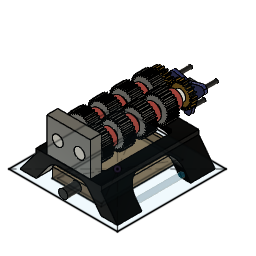
shredder_3d (Autodesk Fusion 360 design; units mm, degrees)
Autodesk Fusion 360 part; units mm, degrees
(part 1 of 2)
sketch "plane" plane through (0, 0, 0) normal (0, 0, 1) x (1, 0, 0)
  line L0 (100, 100) -> (-100, 100)
  line L1 (-100, 100) -> (-100, -100)
  line L2 (-100, -100) -> (100, -100)
  line L3 (100, -100) -> (100, 100)
  line L4 (100, 100) -> (-100, -100) construction
  line L5 (-100, 100) -> (100, -100) construction
  dimension "d1" = 200
  dimension "d2" = 200
  constraint horizontal L0
  constraint perpendicular L0 L1
  constraint parallel L0 L2
  constraint parallel L1 L3
  constraint coincident L4 origin
  constraint coincident L5 origin
  measures "d1" distance of L1.end L2.end
  measures "d2" distance of L0.end L1.end
sketch "holder" plane through (0, 0, 0) normal (0, 1, 0) x (1, 0, 0)
  line L0 (90, 0, 90) -> (60, -40, 90)
  line L1 (60, -40, 90) -> (30, -40, 90)
  line L2 (30, -40, 90) -> (60, 0, 90)
  line L3 (60, 0, 90) -> (90, 0, 90)
  line L4 (0, -30) -> (0, 30)
  line L5 (-30, -40, 90) -> (-60, 0, 90)
  line L6 (-60, -40, 90) -> (-30, -40, 90)
  line L7 (-90, 0, 90) -> (-60, -40, 90)
  line L8 (-60, 0, 90) -> (-90, 0, 90)
  line L9 (30, -40, -90) -> (60, 0, -90)
  line L10 (60, -40, -90) -> (30, -40, -90)
  line L11 (90, 0, -90) -> (60, -40, -90)
  line L12 (60, 0, -90) -> (90, 0, -90)
  line L13 (-60, 0, -90) -> (-90, 0, -90)
  line L14 (-90, 0, -90) -> (-60, -40, -90)
  line L15 (-60, -40, -90) -> (-30, -40, -90)
  line L16 (-30, -40, -90) -> (-60, 0, -90)
  constraint vertical L4
extrude "Extrude1" add sketch "holder" along normal blind 25 contours L9 L10 L11 L12 | L13 L14 L15 L16 in plane through (0, -90, 0) normal (0, 1, 0) makes body 1 at (80, -81.6667, 13.3333) makes body 2 at (-80, -81.6667, 13.3333)
extrude "Extrude2" add sketch "holder" against normal blind 25 separate body contours L0 L1 L2 L3 | L5 L6 L7 L8 in plane through (0, 90, 0) normal (0, 1, 0) makes body 3 at (-80, 81.6667, 13.3333) makes body 4 at (80, 81.6667, 13.3333)
copy_body "Body->Comp1" bodies 1 removing the originals makes body 5 in component "holder_"
copy_body "CutPasteBodies1" bodies 2 removing the originals makes body 6 in component "holder_"
copy_body "CutPasteBodies2" bodies 3 removing the originals makes body 7 in component "holder_"
copy_body "CutPasteBodies3" bodies 4 removing the originals makes body 8 in component "holder_"
sketch "holder_1" plane through (0, 65, 0) normal (0, -1, 0) x (1, 0, 0) in component "holder_"
  line L0 (-90, 0) -> (-60, 0)
  line L1 (-60, 0) -> (-30, 40)
  line L2 (-30, 40) -> (-60, 40)
  line L3 (-60, 40) -> (-90, 0)
  line L4 (-60, 40) -> (-45, 40)
  line L5 (-60, 40) -> (-40, 40)
  line L6 (-60, 40) -> (-90, 0)
  line L7 (-90, 0) -> (-70, 0)
  line L8 (-70, 0) -> (-40, 40)
  line L9 (60, 40) -> (40, 40)
  line L10 (40, 40) -> (70, 0)
  line L11 (70, 0) -> (90, 0)
  line L12 (90, 0) -> (60, 40)
  constraint coincident L2.end L3.start
  constraint midpoint L2 L4.end
  constraint coincident L2 L5.end
  constraint parallel L2 L5
  constraint coincident L0.start L3.end
  constraint coincident L0 L7.end
  constraint parallel L0 L7
  constraint parallel L6 L8
  constraint parallel L0 L9
  constraint parallel L9 L11
  constraint parallel L10 L12
extrude "Extrude1'" add sketch "holder_1" along normal blind 20 contours L0 L2 L3 L4 L5 L6 L7 L8 | L9 L10 L11 L12 bodies 8 makes body 9 at (-70, 58.3333, 26.6667) in component "holder_"
combine "Combine1" operation add target body 9 tool bodies 7 in component "holder_"
sketch "holder_2_extrude" plane through (0, -65, 0) normal (0, 1, 0) x (-1, 0, 0) in component "holder_"
  line L0 (-60, 0) -> (-30, 40)
  line L1 (-30, 40) -> (-60, 40)
  line L2 (-60, 40) -> (-90, 0)
  line L3 (-90, 0) -> (-60, 0)
  line L4 (-60, 40) -> (-40, 40)
  line L5 (-60, 40) -> (-90, 0)
  line L6 (-90, 0) -> (-70, 0)
  line L7 (-70, 0) -> (-40, 40)
  line L8 (60, 40) -> (40, 40)
  line L9 (40, 40) -> (70, 0)
  line L10 (70, 0) -> (90, 0)
  line L11 (90, 0) -> (60, 40)
  constraint coincident L1.end L2.start
  constraint coincident L1 L4.end
  constraint parallel L1 L4
  constraint coincident L2.end L3.start
  constraint coincident L3 L6.end
  constraint parallel L3 L8
  constraint parallel L8 L10
  constraint parallel L9 L11
extrude "Extrude2'" add sketch "holder_2_extrude" along normal blind 20 contours L1 L2 L3 L4 L5 L6 L7 | L8 L9 L10 L11 bodies 5 6 in component "holder_"
sketch "base" plane through (0, 0, 40) normal (0, 0, 1) x (-1, 0, 0) in component "holder_"
  line L0 (60, -90) -> (60, -45)
  line L1 (60, -45) -> (40, -45)
  line L2 (40, -45) -> (40, -65)
  line L3 (40, -65) -> (30, -65)
  line L4 (30, -65) -> (30, -90)
  line L5 (30, -90) -> (60, -90)
  line L6 (60, -90) -> (-60, -90)
  line L7 (-60, -90) -> (-60, -65)
  line L8 (-60, -65) -> (60, -65)
  line L9 (60, -65) -> (60, 90)
  line L10 (60, 90) -> (40, 90)
  line L11 (40, 90) -> (40, -65)
  line L12 (-39.8261, -65) -> (-39.8261, 90)
  line L13 (-39.8261, 90) -> (-60, 90)
  line L14 (-60, 90) -> (-60, -65)
  line L15 (40, 90) -> (-39.8261, 90)
  line L16 (40, 65.705) -> (-39.8261, 65.705)
  constraint coincident L0.start L5.end
  constraint perpendicular L0 L6
  constraint perpendicular L5 L7
  constraint coincident L0 L8.end
  constraint perpendicular L0 L8
  constraint perpendicular L8 L9
  constraint perpendicular L0 L10
  constraint coincident L2.end L3.start
  constraint perpendicular L3 L11
  constraint coincident L8 L12.start
  constraint perpendicular L8 L12
  constraint perpendicular L12 L13
  constraint perpendicular L8 L14
  constraint perpendicular L11 L15
  constraint coincident L11 L16.start
  constraint coincident L12 L16.end
  constraint perpendicular L12 L16
extrude "Extrude3" add sketch "base" along normal blind 8 contours L0 L3 L4 L5 L6 L8 | L0 L1 L2 L8 L9 L11 | L4 L6 L7 L8 | L1 L9 L10 L11 | L8 L12 L13 L14 | L11 L12 L15 L16 bodies 5 6 8 9 in component "holder_"
fillet "Fillet1" radius 24.5 8 edges at (30, 77.5, 40) (50, 45, 40) (50, -45, 40) (30, -77.8525, 40) (-50, 45, 40) (-30, 77.5, 40) (-50, -45, 40) (-30, -77.8525, 40) on bodies 5 in component "holder_"
sketch "decorative_glass" plane through (0, 45, 0) normal (0, -1, 0) x (1, 0, 0) in component "holder_"
  line L0 (78.375, 15.5) -> (58.375, 15.5)
  line L1 (58.375, 15.5) -> (70, 0)
  line L2 (70, 0) -> (90, 0)
  line L3 (90, 0) -> (78.375, 15.5)
  circle A0 centre (75.5122, 6.7743) radius 5
  circle A1 centre (-74.4878, 6.7743) radius 5
  dimension "d15" = 10
  dimension "d16" = 10
  measures "d15" diameter of A0
  measures "d16" diameter of A1
extrude "Extrude4" cut sketch "decorative_glass" along normal blind 100 and the other way blind 20 contours A0 | A1 bodies 5 in component "holder_"
chamfer "Chamfer1" distance 5 angle 45 4 edges at (39.8261, -65.705, 44) (-40, -65.705, 44) (-40, 65, 44) (39.8261, 65, 44) on bodies 5 in component "holder_"
sketch "decorative_glass (1)" plane through (0, -45, 0) normal (0, 1, 0) x (-1, 0, 0) in component "holder_"
  circle A0 centre (-75.5122, 6.7743) radius 5
  line L0 (-58.375, 15.5) -> (-78.375, 15.5)
  line L1 (-78.375, 15.5) -> (-90, 0)
  line L2 (-90, 0) -> (-70, 0)
  line L3 (-70, 0) -> (-58.375, 15.5)
  circle A1 centre (-75.5122, 6.7743) radius 4.85
  circle A2 centre (74.4878, 6.7743) radius 4.85
  dimension "d22" = 9.7
  dimension "d23" = 9.7
  constraint concentric A0 A1
  measures "d22" diameter of A1
  measures "d23" diameter of A2
extrude "Extrude5" add sketch "decorative_glass (1)" along normal blind 105 and the other way blind 5 separate body contours A1 | A2 makes body 10 at (70.6863, 25, 6.2914) makes body 11 at (-79.3137, 25, 6.2914) in component "holder_"
copy_body "Body->Comp1'" bodies 10 removing the originals makes body 12 in component "decoration"
copy_body "CutPasteBodies1'" bodies 11 removing the originals makes body 13 in component "decoration"
sketch "trashbin" plane through (0, 0, 0) normal (0, 0, 1) x (1, 0, 0)
  line L0 (45, 75) -> (-45, 75)
  line L1 (-45, 75) -> (-45, -75)
  line L2 (-45, -75) -> (45, -75)
  line L3 (45, -75) -> (45, 75)
  line L4 (45, 75) -> (-45, -75) construction
  line L5 (-45, 75) -> (45, -75) construction
  line L6 (-40.0498, -70.0498) -> (40.0498, -70.0498)
  line L7 (40.0498, -70.0498) -> (40.0498, 70.0498)
  line L8 (40.0498, 70.0498) -> (-40.0498, 70.0498)
  line L9 (-40.0498, 70.0498) -> (-40.0498, -70.0498)
  dimension "d28" = 90
  dimension "d29" = 150
  dimension "d30" = -4.9502
  constraint horizontal L0
  constraint perpendicular L0 L1
  constraint parallel L0 L2
  constraint parallel L1 L3
  constraint coincident L4 origin
  constraint coincident L5 origin
  measures "d28" distance of L1.end L2.end
  measures "d29" distance of L0.end L1.end
extrude "Extrude3'" add sketch "trashbin" along normal blind 19 separate body makes body 14
extrude "Extrude4'" add sketch "trashbin" along normal blind 5 contours L6 L7 L8 L9 bodies 14
copy_body "Body->Comp2" bodies 14 removing the originals makes body 15 in component "trashbin_removeable"
sketch "handle_sketch" plane through (0, -75, 0) normal (0, -1, 0) x (1, 0, 0) in component "trashbin_removeable"
  line L0 (-45, 0) -> (45, 0)
  line L1 (45, 0) -> (45, 19)
  line L2 (45, 19) -> (-45, 19)
  line L3 (-45, 19) -> (-45, 0)
  circle A0 centre (0, 10) radius 8.3009
extrude "Extrude1''" add sketch "handle_sketch" along normal blind 25 separate body contours A0 makes body 16 in component "trashbin_removeable"
sketch "back_wall" plane through (0, 0, 0) normal (0, 1, 0) x (1, 0, 0) in component "shredder_upperbody"
  line L0 (-40, -48.5, -70) -> (40, -48.5, -70)
  line L1 (40, -48.5, -70) -> (40, -111.5, -70)
  line L2 (40, -111.5, -70) -> (-40, -111.5, -70)
  line L3 (-40, -111.5, -70) -> (-40, -48.5, -70)
  line L4 (-40, -48.5, -70) -> (40, -111.5, -70) construction
  line L5 (40, -48.5, -70) -> (-40, -111.5, -70) construction
  line L6 (0, -111.5, -70) -> (0, -48.5, -70)
  line L7 (-40, -80, -70) -> (-20, -80, -70)
  line L8 (40, -80, -70) -> (20, -80, -70)
  circle A0 through (-10, -80, -70) (-25, -71.3397, -70) (-25, -88.6603, -70)
  circle A1 through (30, -80, -70) (15, -71.3397, -70) (15, -88.6603, -70)
  point P0 (0, -80)
  dimension "d37" = 63
  dimension "d38" = 20
extrude "Extrude1'''" add sketch "back_wall" along normal blind -20 and the other way blind 0 separate body contours L0 L2 L3 L6 | L0 L1 L2 L6 in plane through (0, -70, 0) normal (0, 1, 0) makes body 17 in component "shredder_upperbody"
sketch "pin" plane through (0, 0, 0) normal (0, 1, 0) x (1, 0, 0) in component "blades_2"
  circle A0 centre (-20, -80) radius 9.795
  dimension "d43" = 19.59
  measures "d43" diameter of A0
extrude "Extrude1''''" add sketch "pin" along normal blind 90 and the other way blind 90 separate body makes body 18 in component "blades_2"
sketch "blade_sketch" plane through (0, 90, 0) normal (0, 1, 0) x (-1, 0, 0) in component "blades_2"
  circle A0 centre (20, 80) radius 9.795
  line L0 (16.7621, 104.7894) -> (18.3025, 102.5385)
  line L1 (18.3025, 102.5385) -> (17.1562, 102.2564)
  spline S0 degree 2 poles (17.1562, 102.2564) (16.2391, 98.8702) (14.8092, 101.6787) knots 0 0 0 0.491488 0.491488 0.491488 weights 1 2.231964 1
  line L2 (14.8092, 101.6787) -> (14.1792, 102.916)
  spline S1 degree 2 poles (12.2749, 101.0655) (12.1343, 97.5602) (10.1154, 99.9801) knots 0 0 0 0.491488 0.491488 0.491488 weights 1 2.231964 1
  line L3 (10.1154, 99.9801) -> (9.2259, 101.0462)
  line L4 (11.3271, 103.4474) -> (13.3298, 101.5957)
  line L5 (13.3298, 101.5957) -> (12.2749, 101.0655)
  spline S2 degree 2 poles (7.7811, 98.8184) (8.424, 95.3697) (5.9173, 97.2796) knots 0 0 0 0.491488 0.491488 0.491488 weights 1 2.231964 1
  line L6 (5.9173, 97.2796) -> (4.8128, 98.1211)
  line L7 (6.327, 100.9296) -> (8.6915, 99.57)
  line L8 (8.6915, 99.57) -> (7.7811, 98.8184)
  spline S3 degree 2 poles (3.9, 95.6276) (5.2942, 92.4084) (2.4253, 93.7127) knots 0 0 0 0.491488 0.491488 0.491488 weights 1 2.231964 1
  line L9 (2.4253, 93.7127) -> (1.1612, 94.2873)
  line L10 (2.0125, 97.3624) -> (4.6203, 96.563)
  line L11 (4.6203, 96.563) -> (3.9, 95.6276)
  spline S4 degree 2 poles (0.8262, 91.6532) (2.9018, 88.825) (-0.1854, 89.4581) knots 0 0 0 0.491488 0.491488 0.491488 weights 1 2.231964 1
  line L12 (-0.1854, 89.4581) -> (-1.5457, 89.7371)
  line L13 (-1.4, 92.9245) -> (1.3203, 92.7254)
  line L14 (1.3203, 92.7254) -> (0.8262, 91.6532)
  spline S5 degree 2 poles (-1.2862, 87.0945) (1.3667, 84.799) (-1.784, 84.7293) knots 0 0 0 0.491488 0.491488 0.491488 weights 1 2.231964 1
  line L15 (-1.784, 84.7293) -> (-3.1722, 84.6986)
  line L16 (-3.7394, 87.8385) -> (-1.043, 88.2497)
  line L17 (-1.043, 88.2497) -> (-1.2862, 87.0945)
  spline S6 degree 2 poles (-2.3312, 82.18) (0.766, 80.5324) (-2.2902, 79.7633) knots 0 0 0 0.491488 0.491488 0.491488 weights 1 2.231964 1
  line L18 (-2.2902, 79.7633) -> (-3.6367, 79.4245)
  line L19 (-4.8884, 82.3594) -> (-2.3512, 83.3603)
  line L20 (-2.3512, 83.3603) -> (-2.3312, 82.18)
  spline S7 degree 2 poles (-2.2564, 77.1562) (1.1298, 76.2391) (-1.6787, 74.8092) knots 0 0 0 0.491488 0.491488 0.491488 weights 1 2.231964 1
  line L21 (-1.6787, 74.8092) -> (-2.916, 74.1792)
  line L22 (-4.7894, 76.7621) -> (-2.5385, 78.3025)
  line L23 (-2.5385, 78.3025) -> (-2.2564, 77.1562)
  spline S8 degree 2 poles (-1.0655, 72.2749) (2.4398, 72.1343) (0.0199, 70.1154) knots 0 0 0 0.491488 0.491488 0.491488 weights 1 2.231964 1
  line L24 (0.0199, 70.1154) -> (-1.0462, 69.2259)
  line L25 (-3.4474, 71.3271) -> (-1.5957, 73.3298)
  line L26 (-1.5957, 73.3298) -> (-1.0655, 72.2749)
  spline S9 degree 2 poles (1.1816, 67.7811) (4.6303, 68.424) (2.7204, 65.9173) knots 0 0 0 0.491488 0.491488 0.491488 weights 1 2.231964 1
  line L27 (2.7204, 65.9173) -> (1.8789, 64.8128)
  line L28 (-0.9296, 66.327) -> (0.43, 68.6915)
  line L29 (0.43, 68.6915) -> (1.1816, 67.7811)
  spline S10 degree 2 poles (4.3724, 63.9) (7.5916, 65.2942) (6.2873, 62.4253) knots 0 0 0 0.491488 0.491488 0.491488 weights 1 2.231964 1
  line L30 (6.2873, 62.4253) -> (5.7127, 61.1612)
  line L31 (2.6376, 62.0125) -> (3.437, 64.6203)
  line L32 (3.437, 64.6203) -> (4.3724, 63.9)
  spline S11 degree 2 poles (8.3468, 60.8262) (11.175, 62.9018) (10.5419, 59.8146) knots 0 0 0 0.491488 0.491488 0.491488 weights 1 2.231964 1
  line L33 (10.5419, 59.8146) -> (10.2629, 58.4543)
  line L34 (7.0755, 58.6) -> (7.2746, 61.3203)
  line L35 (7.2746, 61.3203) -> (8.3468, 60.8262)
  spline S12 degree 2 poles (12.9055, 58.7138) (15.201, 61.3667) (15.2707, 58.216) knots 0 0 0 0.491488 0.491488 0.491488 weights 1 2.231964 1
  line L36 (15.2707, 58.216) -> (15.3014, 56.8278)
  line L37 (12.1615, 56.2606) -> (11.7503, 58.957)
  line L38 (11.7503, 58.957) -> (12.9055, 58.7138)
  spline S13 degree 2 poles (17.82, 57.6688) (19.4676, 60.766) (20.2367, 57.7098) knots 0 0 0 0.491488 0.491488 0.491488 weights 1 2.231964 1
  line L39 (20.2367, 57.7098) -> (20.5755, 56.3633)
  line L40 (17.6406, 55.1116) -> (16.6397, 57.6488)
  line L41 (16.6397, 57.6488) -> (17.82, 57.6688)
  spline S14 degree 2 poles (22.8438, 57.7436) (23.7609, 61.1298) (25.1908, 58.3213) knots 0 0 0 0.491488 0.491488 0.491488 weights 1 2.231964 1
  line L42 (25.1908, 58.3213) -> (25.8208, 57.084)
  line L43 (23.2379, 55.2106) -> (21.6975, 57.4615)
  line L44 (21.6975, 57.4615) -> (22.8438, 57.7436)
  spline S15 degree 2 poles (27.7251, 58.9345) (27.8657, 62.4398) (29.8846, 60.0199) knots 0 0 0 0.491488 0.491488 0.491488 weights 1 2.231964 1
  line L45 (29.8846, 60.0199) -> (30.7741, 58.9538)
  line L46 (28.6729, 56.5526) -> (26.6702, 58.4043)
  line L47 (26.6702, 58.4043) -> (27.7251, 58.9345)
  spline S16 degree 2 poles (32.2189, 61.1816) (31.576, 64.6303) (34.0827, 62.7204) knots 0 0 0 0.491488 0.491488 0.491488 weights 1 2.231964 1
  line L48 (34.0827, 62.7204) -> (35.1872, 61.8789)
  line L49 (33.673, 59.0704) -> (31.3085, 60.43)
  line L50 (31.3085, 60.43) -> (32.2189, 61.1816)
  spline S17 degree 2 poles (36.1, 64.3724) (34.7058, 67.5916) (37.5747, 66.2873) knots 0 0 0 0.491488 0.491488 0.491488 weights 1 2.231964 1
  line L51 (37.5747, 66.2873) -> (38.8388, 65.7127)
  line L52 (37.9875, 62.6376) -> (35.3797, 63.437)
  line L53 (35.3797, 63.437) -> (36.1, 64.3724)
  spline S18 degree 2 poles (39.1738, 68.3468) (37.0982, 71.175) (40.1854, 70.5419) knots 0 0 0 0.491488 0.491488 0.491488 weights 1 2.231964 1
  line L54 (40.1854, 70.5419) -> (41.5457, 70.2629)
  line L55 (41.4, 67.0755) -> (38.6797, 67.2746)
  line L56 (38.6797, 67.2746) -> (39.1738, 68.3468)
  spline S19 degree 2 poles (41.2862, 72.9055) (38.6333, 75.201) (41.784, 75.2707) knots 0 0 0 0.491488 0.491488 0.491488 weights 1 2.231964 1
  line L57 (41.784, 75.2707) -> (43.1722, 75.3014)
  line L58 (43.7394, 72.1615) -> (41.043, 71.7503)
  line L59 (41.043, 71.7503) -> (41.2862, 72.9055)
  spline S20 degree 2 poles (42.3312, 77.82) (39.234, 79.4676) (42.2902, 80.2367) knots 0 0 0 0.491488 0.491488 0.491488 weights 1 2.231964 1
  line L60 (42.2902, 80.2367) -> (43.6367, 80.5755)
  line L61 (44.8884, 77.6406) -> (42.3512, 76.6397)
  line L62 (42.3512, 76.6397) -> (42.3312, 77.82)
  spline S21 degree 2 poles (42.2564, 82.8438) (38.8702, 83.7609) (41.6787, 85.1908) knots 0 0 0 0.491488 0.491488 0.491488 weights 1 2.231964 1
  line L63 (41.6787, 85.1908) -> (42.916, 85.8208)
  line L64 (44.7894, 83.2379) -> (42.5385, 81.6975)
  line L65 (42.5385, 81.6975) -> (42.2564, 82.8438)
  spline S22 degree 2 poles (41.0655, 87.7251) (37.5602, 87.8657) (39.9801, 89.8846) knots 0 0 0 0.491488 0.491488 0.491488 weights 1 2.231964 1
  line L66 (39.9801, 89.8846) -> (41.0462, 90.7741)
  line L67 (43.4474, 88.6729) -> (41.5957, 86.6702)
  line L68 (41.5957, 86.6702) -> (41.0655, 87.7251)
  spline S23 degree 2 poles (38.8184, 92.2189) (35.3697, 91.576) (37.2796, 94.0827) knots 0 0 0 0.491488 0.491488 0.491488 weights 1 2.231964 1
  line L69 (37.2796, 94.0827) -> (38.1211, 95.1872)
  line L70 (40.9296, 93.673) -> (39.57, 91.3085)
  line L71 (39.57, 91.3085) -> (38.8184, 92.2189)
  spline S24 degree 2 poles (35.6276, 96.1) (32.4084, 94.7058) (33.7127, 97.5747) knots 0 0 0 0.491488 0.491488 0.491488 weights 1 2.231964 1
  line L72 (33.7127, 97.5747) -> (34.2873, 98.8388)
  line L73 (37.3624, 97.9875) -> (36.563, 95.3797)
  line L74 (36.563, 95.3797) -> (35.6276, 96.1)
  spline S25 degree 2 poles (31.6532, 99.1738) (28.825, 97.0982) (29.4581, 100.1854) knots 0 0 0 0.491488 0.491488 0.491488 weights 1 2.231964 1
  line L75 (29.4581, 100.1854) -> (29.7371, 101.5457)
  line L76 (32.9245, 101.4) -> (32.7254, 98.6797)
  line L77 (32.7254, 98.6797) -> (31.6532, 99.1738)
  spline S26 degree 2 poles (27.0945, 101.2862) (24.799, 98.6333) (24.7293, 101.784) knots 0 0 0 0.491488 0.491488 0.491488 weights 1 2.231964 1
  line L78 (24.7293, 101.784) -> (24.6986, 103.1722)
  line L79 (27.8385, 103.7394) -> (28.2497, 101.043)
  line L80 (28.2497, 101.043) -> (27.0945, 101.2862)
  spline S27 degree 2 poles (22.18, 102.3312) (20.5324, 99.234) (19.7633, 102.2902) knots 0 0 0 0.491488 0.491488 0.491488 weights 1 2.231964 1
  line L81 (19.7633, 102.2902) -> (19.4245, 103.6367)
  line L82 (22.3594, 104.8884) -> (23.3603, 102.3512)
  line L83 (23.3603, 102.3512) -> (22.18, 102.3312)
  line L84 (11.3271, 103.4474) -> (14.1792, 102.916)
  line L85 (6.327, 100.9296) -> (9.2259, 101.0462)
  line L86 (2.0125, 97.3624) -> (4.8128, 98.1211)
  line L87 (-1.4, 92.9245) -> (1.1612, 94.2873)
  line L88 (-3.7394, 87.8385) -> (-1.5457, 89.7371)
  line L89 (-4.8884, 82.3594) -> (-3.1722, 84.6986)
  line L90 (-4.7894, 76.7621) -> (-3.6367, 79.4245)
  line L91 (-3.4474, 71.3271) -> (-2.916, 74.1792)
  line L92 (-0.9296, 66.327) -> (-1.0462, 69.2259)
  line L93 (2.6376, 62.0125) -> (1.8789, 64.8128)
  line L94 (7.0755, 58.6) -> (5.7127, 61.1612)
  line L95 (12.1615, 56.2606) -> (10.2629, 58.4543)
  line L96 (17.6406, 55.1116) -> (15.3014, 56.8278)
  line L97 (23.2379, 55.2106) -> (20.5755, 56.3633)
  line L98 (28.6729, 56.5526) -> (25.8208, 57.084)
  line L99 (33.673, 59.0704) -> (30.7741, 58.9538)
  line L100 (37.9875, 62.6376) -> (35.1872, 61.8789)
  line L101 (41.4, 67.0755) -> (38.8388, 65.7127)
  line L102 (43.7394, 72.1615) -> (41.5457, 70.2629)
  line L103 (44.8884, 77.6406) -> (43.1722, 75.3014)
  line L104 (44.7894, 83.2379) -> (43.6367, 80.5755)
  line L105 (43.4474, 88.6729) -> (42.916, 85.8208)
  line L106 (40.9296, 93.673) -> (41.0462, 90.7741)
  line L107 (37.3624, 97.9875) -> (38.1211, 95.1872)
  line L108 (32.9245, 101.4) -> (34.2873, 98.8388)
  line L109 (27.8385, 103.7394) -> (29.7371, 101.5457)
  line L110 (22.3594, 104.8884) -> (24.6986, 103.1722)
  line L111 (16.7621, 104.7894) -> (19.4245, 103.6367)
extrude "Extrude2''" add sketch "blade_sketch" against normal blind 20 separate body makes body 19 in component "blades_2"
fillet "Fillet1'" radius 0.5 28 edges at (-14.1792, 80, 102.916) (-19.4245, 80, 103.6367) (-24.6986, 80, 103.1722) (-29.7371, 80, 101.5457) (-34.2873, 80, 98.8388) (-38.1211, 80, 95.1872) (-41.0462, 80, 90.7741) (-42.916, 80, 85.8208) (-43.6367, 80, 80.5755) (-43.1722, 80, 75.3014) (-41.5457, 80, 70.2629) (-38.8388, 80, 65.7127) (-35.1872, 80, 61.8789) (-30.7741, 80, 58.9538) (-25.8208, 80, 57.084) (-20.5755, 80, 56.3633) (-15.3014, 80, 56.8278) (-10.2629, 80, 58.4543) (-5.7127, 80, 61.1612) (-1.8789, 80, 64.8128) (1.0462, 80, 69.2259) (2.916, 80, 74.1792) (3.6367, 80, 79.4245) (3.1722, 80, 84.6986) (1.5457, 80, 89.7371) (-1.1612, 80, 94.2873) (-4.8128, 80, 98.1211) (-9.2259, 80, 101.0462) on bodies 19 in component "blades_2"
copy_body "CopyPasteBodies1" bodies 19 makes body 20 in component "blades_2"
move_body "Move1" bodies 20 to x (1, 0, 0) y (0, 1, 0) z (0, 0, 1) at (0, -40, 0) in component "blades_2"
copy_body "CopyPasteBodies2" bodies 20 makes body 21 in component "blades_2"
move_body "Move2" bodies 21 to x (1, 0, 0) y (0, 1, 0) z (0, 0, 1) at (0, -40, 0) in component "blades_2"
copy_body "CopyPasteBodies3" bodies 21 makes body 22 in component "blades_2"
move_body "Move3" bodies 22 to x (1, 0, 0) y (0, 1, 0) z (0, 0, 1) at (0, -40, 0) in component "blades_2"
sketch "blade_replacement" plane through (0, 0, 0) normal (0, 1, 0) x (1, 0, 0) in component "blades_2"
  circle A0 through (-5, -80, 15) (-27.5, -67.0096, 15) (-27.5, -92.9904, 15)
  circle A1 through (-10, -80, 15) (-25, -71.3397, 15) (-25, -88.6603, 15)
  dimension "d58" = 30
  dimension "d59" = 20
extrude "Extrude3''" add sketch "blade_replacement" along normal blind 10 separate body contours A0 in plane through (0, 15, 0) normal (0, 1, 0) makes body 23 in component "blades_2"
copy_body "CopyPasteBodies4" bodies 23 makes body 24 in component "blades_2"
move_body "Move4" bodies 24 to x (1, 0, 0) y (0, 1, 0) z (0, 0, 1) at (0, 40, 0) in component "blades_2"
copy_body "CopyPasteBodies5" bodies 23 makes body 25 in component "blades_2"
move_body "Move5" bodies 25 to x (1, 0, 0) y (0, 1, 0) z (0, 0, 1) at (0, -40, 0) in component "blades_2"
copy_body "CopyPasteBodies6" bodies 25 makes body 26 in component "blades_2"
move_body "Move6" bodies 26 to x (1, 0, 0) y (0, 1, 0) z (0, 0, 1) at (0, -40, 0) in component "blades_2"
copy_body "CopyPasteBodies1'" bodies 19 makes body 27
move_body "Move1'" bodies 27 to x (1, 0, 0) y (0, 1, 0) z (0, 0, 1) at (40, -20, 0)
copy_body "CutPasteBodies1''" bodies 27 removing the originals makes body 28 in component "blades_1"
sketch "pin_sketch" plane through (0, -70, 0) normal (0, 1, 0) x (-1, 0, 0) in component "blades_1"
  circle A0 centre (20, 80) radius 10
  circle A1 centre (-20, 80) radius 10
  line L0 (40, 111.5) -> (-40, 111.5)
  line L1 (-40, 111.5) -> (-40, 48.5)
  line L2 (-40, 48.5) -> (40, 48.5)
  line L3 (40, 48.5) -> (40, 111.5)
  circle A2 centre (-20, 80) radius 9.9
  dimension "d62" = 19.8
  constraint concentric A1 A2
  measures "d62" diameter of A2
extrude "Extrude1'''''" add sketch "pin_sketch" along normal blind 185 and the other way blind 20 separate body contours A2 makes body 29 in component "blades_1"
sketch "Sketch2" plane through (0, 50, 0) normal (0, -1, 0) x (1, 0, 0) in component "blades_1"
  arc A0 (31.0203, 101.0363) -> (30.6163, 100.8571) centre (31.0002, 100.5367) ccw
  line L0 (30.6163, 100.8571) -> (29.8846, 99.9801)
  spline S0 degree 2 poles (29.8846, 99.9801) (27.8657, 97.5602) (27.7251, 101.0655) knots -0.491488 -0.491488 -0.491488 0 0 0 weights 1 2.231964 1
  line L1 (27.7251, 101.0655) -> (26.6702, 101.5957)
  line L2 (26.6702, 101.5957) -> (28.6729, 103.4474)
  line L3 (28.6729, 103.4474) -> (26.063, 102.9612)
  arc A1 (26.063, 102.9612) -> (25.709, 102.6965) centre (26.1545, 102.4696) ccw
  line L4 (25.709, 102.6965) -> (25.1908, 101.6787)
  spline S1 degree 2 poles (25.1908, 101.6787) (23.7609, 98.8702) (22.8438, 102.2564) knots -0.491488 -0.491488 -0.491488 0 0 0 weights 1 2.231964 1
  line L5 (22.8438, 102.2564) -> (21.6975, 102.5385)
  line L6 (21.6975, 102.5385) -> (23.2379, 104.7894)
  line L7 (23.2379, 104.7894) -> (20.8016, 103.7346)
  arc A2 (20.8016, 103.7346) -> (20.5154, 103.3978) centre (21.0003, 103.2758) ccw
  line L8 (20.5154, 103.3978) -> (20.2367, 102.2902)
  spline S2 degree 2 poles (20.2367, 102.2902) (19.4676, 99.234) (17.82, 102.3312) knots -0.491488 -0.491488 -0.491488 0 0 0 weights 1 2.231964 1
  line L9 (17.82, 102.3312) -> (16.6397, 102.3512)
  line L10 (16.6397, 102.3512) -> (17.6406, 104.8884)
  line L11 (17.6406, 104.8884) -> (15.5001, 103.3179)
  arc A3 (15.5001, 103.3179) -> (15.296, 102.9258) centre (15.7958, 102.9148) ccw
  line L12 (15.296, 102.9258) -> (15.2707, 101.784)
  spline S3 degree 2 poles (15.2707, 101.784) (15.201, 98.6333) (12.9055, 101.2862) knots -0.491488 -0.491488 -0.491488 0 0 0 weights 1 2.231964 1
  line L13 (12.9055, 101.2862) -> (11.7503, 101.043)
  line L14 (11.7503, 101.043) -> (12.1615, 103.7394)
  line L15 (12.1615, 103.7394) -> (10.4242, 101.732)
  arc A4 (10.4242, 101.732) -> (10.3124, 101.3043) centre (10.8022, 101.4048) ccw
  line L16 (10.3124, 101.3043) -> (10.5419, 100.1854)
  spline S4 degree 2 poles (10.5419, 100.1854) (11.175, 97.0982) (8.3468, 99.1738) knots -0.491488 -0.491488 -0.491488 0 0 0 weights 1 2.231964 1
  line L17 (8.3468, 99.1738) -> (7.2746, 98.6797)
  line L18 (7.2746, 98.6797) -> (7.0755, 101.4)
  line L19 (7.0755, 101.4) -> (5.8284, 99.0563)
  arc A5 (5.8284, 99.0563) -> (5.8147, 98.6145) centre (6.2698, 98.8214) ccw
  line L20 (5.8147, 98.6145) -> (6.2873, 97.5747)
  spline S5 degree 2 poles (6.2873, 97.5747) (7.5916, 94.7058) (4.3724, 96.1) knots -0.491488 -0.491488 -0.491488 0 0 0 weights 1 2.231964 1
  line L21 (4.3724, 96.1) -> (3.437, 95.3797)
  line L22 (3.437, 95.3797) -> (2.6376, 97.9875)
  line L23 (2.6376, 97.9875) -> (1.9433, 95.425)
  arc A6 (1.9433, 95.425) -> (2.0282, 94.9912) centre (2.4259, 95.2943) ccw
  line L24 (2.0282, 94.9912) -> (2.7204, 94.0827)
  spline S6 degree 2 poles (2.7204, 94.0827) (4.6303, 91.576) (1.1816, 92.2189) knots -0.491488 -0.491488 -0.491488 0 0 0 weights 1 2.231964 1
  line L25 (1.1816, 92.2189) -> (0.43, 91.3085)
  line L26 (0.43, 91.3085) -> (-0.9296, 93.673)
  line L27 (-0.9296, 93.673) -> (-1.0363, 91.0203)
  arc A7 (-1.0363, 91.0203) -> (-0.8571, 90.6163) centre (-0.5367, 91.0002) ccw
  line L28 (-0.8571, 90.6163) -> (0.0199, 89.8846)
  spline S7 degree 2 poles (0.0199, 89.8846) (2.4398, 87.8657) (-1.0655, 87.7251) knots -0.491488 -0.491488 -0.491488 0 0 0 weights 1 2.231964 1
  line L29 (-1.0655, 87.7251) -> (-1.5957, 86.6702)
  line L30 (-1.5957, 86.6702) -> (-3.4474, 88.6729)
  line L31 (-3.4474, 88.6729) -> (-2.9612, 86.063)
  arc A8 (-2.9612, 86.063) -> (-2.6965, 85.709) centre (-2.4696, 86.1545) ccw
  line L32 (-2.6965, 85.709) -> (-1.6787, 85.1908)
  spline S8 degree 2 poles (-1.6787, 85.1908) (1.1298, 83.7609) (-2.2564, 82.8438) knots -0.491488 -0.491488 -0.491488 0 0 0 weights 1 2.231964 1
  line L33 (-2.2564, 82.8438) -> (-2.5385, 81.6975)
  line L34 (-2.5385, 81.6975) -> (-4.7894, 83.2379)
  line L35 (-4.7894, 83.2379) -> (-3.7346, 80.8016)
  arc A9 (-3.7346, 80.8016) -> (-3.3978, 80.5154) centre (-3.2758, 81.0003) ccw
  line L36 (-3.3978, 80.5154) -> (-2.2902, 80.2367)
  spline S9 degree 2 poles (-2.2902, 80.2367) (0.766, 79.4676) (-2.3312, 77.82) knots -0.491488 -0.491488 -0.491488 0 0 0 weights 1 2.231964 1
  line L37 (-2.3312, 77.82) -> (-2.3512, 76.6397)
  line L38 (-2.3512, 76.6397) -> (-4.8884, 77.6406)
  line L39 (-4.8884, 77.6406) -> (-3.3179, 75.5001)
  arc A10 (-3.3179, 75.5001) -> (-2.9258, 75.296) centre (-2.9148, 75.7958) ccw
  line L40 (-2.9258, 75.296) -> (-1.784, 75.2707)
  spline S10 degree 2 poles (-1.784, 75.2707) (1.3667, 75.201) (-1.2862, 72.9055) knots -0.491488 -0.491488 -0.491488 0 0 0 weights 1 2.231964 1
  line L41 (-1.2862, 72.9055) -> (-1.043, 71.7503)
  line L42 (-1.043, 71.7503) -> (-3.7394, 72.1615)
  line L43 (-3.7394, 72.1615) -> (-1.732, 70.4242)
  arc A11 (-1.732, 70.4242) -> (-1.3043, 70.3124) centre (-1.4048, 70.8022) ccw
  line L44 (-1.3043, 70.3124) -> (-0.1854, 70.5419)
  spline S11 degree 2 poles (-0.1854, 70.5419) (2.9018, 71.175) (0.8262, 68.3468) knots -0.491488 -0.491488 -0.491488 0 0 0 weights 1 2.231964 1
  line L45 (0.8262, 68.3468) -> (1.3203, 67.2746)
  line L46 (1.3203, 67.2746) -> (-1.4, 67.0755)
  line L47 (-1.4, 67.0755) -> (0.9437, 65.8284)
  arc A12 (0.9437, 65.8284) -> (1.3855, 65.8147) centre (1.1786, 66.2698) ccw
  line L48 (1.3855, 65.8147) -> (2.4253, 66.2873)
  spline S12 degree 2 poles (2.4253, 66.2873) (5.2942, 67.5916) (3.9, 64.3724) knots -0.491488 -0.491488 -0.491488 0 0 0 weights 1 2.231964 1
  line L49 (3.9, 64.3724) -> (4.6203, 63.437)
  line L50 (4.6203, 63.437) -> (2.0125, 62.6376)
  line L51 (2.0125, 62.6376) -> (4.575, 61.9433)
  arc A13 (4.575, 61.9433) -> (5.0088, 62.0282) centre (4.7057, 62.4259) ccw
  line L52 (5.0088, 62.0282) -> (5.9173, 62.7204)
  spline S13 degree 2 poles (5.9173, 62.7204) (8.424, 64.6303) (7.7811, 61.1816) knots -0.491488 -0.491488 -0.491488 0 0 0 weights 1 2.231964 1
  line L53 (7.7811, 61.1816) -> (8.6915, 60.43)
  line L54 (8.6915, 60.43) -> (6.327, 59.0704)
  line L55 (6.327, 59.0704) -> (8.9797, 58.9637)
  arc A14 (8.9797, 58.9637) -> (9.3837, 59.1429) centre (8.9998, 59.4633) ccw
  line L56 (9.3837, 59.1429) -> (10.1154, 60.0199)
  spline S14 degree 2 poles (10.1154, 60.0199) (12.1343, 62.4398) (12.2749, 58.9345) knots -0.491488 -0.491488 -0.491488 0 0 0 weights 1 2.231964 1
  line L57 (12.2749, 58.9345) -> (13.3298, 58.4043)
  line L58 (13.3298, 58.4043) -> (11.3271, 56.5526)
  line L59 (11.3271, 56.5526) -> (13.937, 57.0388)
  arc A15 (13.937, 57.0388) -> (14.291, 57.3035) centre (13.8455, 57.5304) ccw
  line L60 (14.291, 57.3035) -> (14.8092, 58.3213)
  spline S15 degree 2 poles (14.8092, 58.3213) (16.2391, 61.1298) (17.1562, 57.7436) knots -0.491488 -0.491488 -0.491488 0 0 0 weights 1 2.231964 1
  line L61 (17.1562, 57.7436) -> (18.3025, 57.4615)
  line L62 (18.3025, 57.4615) -> (16.7621, 55.2106)
  line L63 (16.7621, 55.2106) -> (19.1984, 56.2654)
  arc A16 (19.1984, 56.2654) -> (19.4846, 56.6022) centre (18.9997, 56.7242) ccw
  line L64 (19.4846, 56.6022) -> (19.7633, 57.7098)
  spline S16 degree 2 poles (19.7633, 57.7098) (20.5324, 60.766) (22.18, 57.6688) knots -0.491488 -0.491488 -0.491488 0 0 0 weights 1 2.231964 1
  line L65 (22.18, 57.6688) -> (23.3603, 57.6488)
  line L66 (23.3603, 57.6488) -> (22.3594, 55.1116)
  line L67 (22.3594, 55.1116) -> (24.4999, 56.6821)
  arc A17 (24.4999, 56.6821) -> (24.704, 57.0742) centre (24.2042, 57.0852) ccw
  line L68 (24.704, 57.0742) -> (24.7293, 58.216)
  spline S17 degree 2 poles (24.7293, 58.216) (24.799, 61.3667) (27.0945, 58.7138) knots -0.491488 -0.491488 -0.491488 0 0 0 weights 1 2.231964 1
  line L69 (27.0945, 58.7138) -> (28.2497, 58.957)
  line L70 (28.2497, 58.957) -> (27.8385, 56.2606)
  line L71 (27.8385, 56.2606) -> (29.5758, 58.268)
  arc A18 (29.5758, 58.268) -> (29.6876, 58.6957) centre (29.1978, 58.5952) ccw
  line L72 (29.6876, 58.6957) -> (29.4581, 59.8146)
  spline S18 degree 2 poles (29.4581, 59.8146) (28.825, 62.9018) (31.6532, 60.8262) knots -0.491488 -0.491488 -0.491488 0 0 0 weights 1 2.231964 1
  line L73 (31.6532, 60.8262) -> (32.7254, 61.3203)
  line L74 (32.7254, 61.3203) -> (32.9245, 58.6)
  line L75 (32.9245, 58.6) -> (34.1716, 60.9437)
  arc A19 (34.1716, 60.9437) -> (34.1853, 61.3855) centre (33.7302, 61.1786) ccw
  line L76 (34.1853, 61.3855) -> (33.7127, 62.4253)
  spline S19 degree 2 poles (33.7127, 62.4253) (32.4084, 65.2942) (35.6276, 63.9) knots -0.491488 -0.491488 -0.491488 0 0 0 weights 1 2.231964 1
  line L77 (35.6276, 63.9) -> (36.563, 64.6203)
  line L78 (36.563, 64.6203) -> (37.3624, 62.0125)
  line L79 (37.3624, 62.0125) -> (38.0567, 64.575)
  arc A20 (38.0567, 64.575) -> (37.9718, 65.0088) centre (37.5741, 64.7057) ccw
  line L80 (37.9718, 65.0088) -> (37.2796, 65.9173)
  spline S20 degree 2 poles (37.2796, 65.9173) (35.3697, 68.424) (38.8184, 67.7811) knots -0.491488 -0.491488 -0.491488 0 0 0 weights 1 2.231964 1
  line L81 (38.8184, 67.7811) -> (39.57, 68.6915)
  line L82 (39.57, 68.6915) -> (40.9296, 66.327)
  line L83 (40.9296, 66.327) -> (41.0363, 68.9797)
  arc A21 (41.0363, 68.9797) -> (40.8571, 69.3837) centre (40.5367, 68.9998) ccw
  line L84 (40.8571, 69.3837) -> (39.9801, 70.1154)
  spline S21 degree 2 poles (39.9801, 70.1154) (37.5602, 72.1343) (41.0655, 72.2749) knots -0.491488 -0.491488 -0.491488 0 0 0 weights 1 2.231964 1
  line L85 (41.0655, 72.2749) -> (41.5957, 73.3298)
  line L86 (41.5957, 73.3298) -> (43.4474, 71.3271)
  line L87 (43.4474, 71.3271) -> (42.9612, 73.937)
  arc A22 (42.9612, 73.937) -> (42.6965, 74.291) centre (42.4696, 73.8455) ccw
  line L88 (42.6965, 74.291) -> (41.6787, 74.8092)
  spline S22 degree 2 poles (41.6787, 74.8092) (38.8702, 76.2391) (42.2564, 77.1562) knots -0.491488 -0.491488 -0.491488 0 0 0 weights 1 2.231964 1
  line L89 (42.2564, 77.1562) -> (42.5385, 78.3025)
  line L90 (42.5385, 78.3025) -> (44.7894, 76.7621)
  line L91 (44.7894, 76.7621) -> (43.7346, 79.1984)
  arc A23 (43.7346, 79.1984) -> (43.3978, 79.4846) centre (43.2758, 78.9997) ccw
  line L92 (43.3978, 79.4846) -> (42.2902, 79.7633)
  spline S23 degree 2 poles (42.2902, 79.7633) (39.234, 80.5324) (42.3312, 82.18) knots -0.491488 -0.491488 -0.491488 0 0 0 weights 1 2.231964 1
  line L93 (42.3312, 82.18) -> (42.3512, 83.3603)
  line L94 (42.3512, 83.3603) -> (44.8884, 82.3594)
  line L95 (44.8884, 82.3594) -> (43.3179, 84.4999)
  arc A24 (43.3179, 84.4999) -> (42.9258, 84.704) centre (42.9148, 84.2042) ccw
  line L96 (42.9258, 84.704) -> (41.784, 84.7293)
  spline S24 degree 2 poles (41.784, 84.7293) (38.6333, 84.799) (41.2862, 87.0945) knots -0.491488 -0.491488 -0.491488 0 0 0 weights 1 2.231964 1
  line L97 (41.2862, 87.0945) -> (41.043, 88.2497)
  line L98 (41.043, 88.2497) -> (43.7394, 87.8385)
  line L99 (43.7394, 87.8385) -> (41.732, 89.5758)
  arc A25 (41.732, 89.5758) -> (41.3043, 89.6876) centre (41.4048, 89.1978) ccw
  line L100 (41.3043, 89.6876) -> (40.1854, 89.4581)
  spline S25 degree 2 poles (40.1854, 89.4581) (37.0982, 88.825) (39.1738, 91.6532) knots -0.491488 -0.491488 -0.491488 0 0 0 weights 1 2.231964 1
  line L101 (39.1738, 91.6532) -> (38.6797, 92.7254)
  line L102 (38.6797, 92.7254) -> (41.4, 92.9245)
  line L103 (41.4, 92.9245) -> (39.0563, 94.1716)
  arc A26 (39.0563, 94.1716) -> (38.6145, 94.1853) centre (38.8214, 93.7302) ccw
  line L104 (38.6145, 94.1853) -> (37.5747, 93.7127)
  spline S26 degree 2 poles (37.5747, 93.7127) (34.7058, 92.4084) (36.1, 95.6276) knots -0.491488 -0.491488 -0.491488 0 0 0 weights 1 2.231964 1
  line L105 (36.1, 95.6276) -> (35.3797, 96.563)
  line L106 (35.3797, 96.563) -> (37.9875, 97.3624)
  line L107 (37.9875, 97.3624) -> (35.425, 98.0567)
  arc A27 (35.425, 98.0567) -> (34.9912, 97.9718) centre (35.2943, 97.5741) ccw
  line L108 (34.9912, 97.9718) -> (34.0827, 97.2796)
  spline S27 degree 2 poles (34.0827, 97.2796) (31.576, 95.3697) (32.2189, 98.8184) knots -0.491488 -0.491488 -0.491488 0 0 0 weights 1 2.231964 1
  line L109 (32.2189, 98.8184) -> (31.3085, 99.57)
  line L110 (31.3085, 99.57) -> (33.673, 100.9296)
  line L111 (33.673, 100.9296) -> (31.0203, 101.0363)
  circle A28 centre (20, 80) radius 9.795
  circle A29 centre (20, 80) radius 25
  constraint concentric A28 A29
  constraint coincident L46.end A29
extrude "Extrude2'''" cut sketch "Sketch2" along normal blind 0 and the other way blind 0.5 contours A0 L0 S0 L1 L2 L3 A1 L4 S1 L5 L6 L7 A2 L8 S2 L9 L10 L11 A3 L12 S3 L13 L14 L15 A4 L16 S4 L17 L18 L19 A5 L20 S5 L21 L22 L23 A6 L24 S6 L25 L26 L27 A7 L28 S7 L29 L30 L31 A8 L32 S8 L33 L34 L35 A9 L36 S9 L37 L38 L39 A10 L40 S10 L41 L42 L43 A11 L44 S11 L45 L46 L47 A12 L48 S12 L49 L50 L51 A13 L52 S13 L53 L54 L55 A14 L56 S14 L57 L58 L59 A15 L60 S15 L61 L62 L63 A16 L64 S16 L65 L66 L67 A17 L68 S17 L69 L70 L71 A18 L72 S18 L73 L74 L75 A19 L76 S19 L77 L78 L79 A20 L80 S20 L81 L82 L83 A21 L84 S21 L85 L86 L87 A22 L88 S22 L89 L90 L91 A23 L92 S23 L93 L94 L95 A24 L96 S24 L97 L98 L99 A25 L100 S25 L101 L102 L103 A26 L104 S26 L105 L106 L107 A27 L108 S27 L109 L110 L111 bodies 28 in component "blades_1"
move_body "Move1''" bodies 28 to x (1, 0, 0) y (0, 1, 0) z (0, 0, 1) at (0, -0.5, 0) in component "blades_1"
move_body "Move2'" bodies 28 to x (1, 0, 0) y (0, 1, 0) z (0, 0, 1) at (0, -120, 0) in component "blades_1"
copy_body "CopyPasteBodies2'" bodies 28 makes body 30 in component "blades_1"
move_body "Move3'" bodies 30 to x (1, 0, 0) y (0, 1, 0) z (0, 0, 1) at (0, 40, 0) in component "blades_1"
copy_body "CopyPasteBodies3'" bodies 30 makes body 31 in component "blades_1"
move_body "Move4'" bodies 31 to x (1, 0, 0) y (0, 1, 0) z (0, 0, 1) at (0, 40, 0) in component "blades_1"
copy_body "CopyPasteBodies4'" bodies 31 makes body 32 in component "blades_1"
move_body "Move5'" bodies 32 to x (1, 0, 0) y (0, 1, 0) z (0, 0, 1) at (0, 40, 0) in component "blades_1"
sketch "blade_replace" plane through (0, 0, 0) normal (0, 1, 0) x (1, 0, 0) in component "blades_1"
  circle A0 through (34.75, -80, 56) (12.625, -67.2261, 56) (12.625, -92.7739, 56)
  dimension "d71" = 29.5
extrude "Extrude3'''" add sketch "blade_replace" along normal blind 10 separate body contours A0 in plane through (0, 56, 0) normal (0, 1, 0) makes body 33 in component "blades_1"
move_body "Move6'" bodies 33 to x (1, 0, 0) y (0, 1, 0) z (0, 0, 1) at (0, 20, 0) in component "blades_1"
copy_body "CopyPasteBodies5'" bodies 33 makes body 34 in component "blades_1"
move_body "Move7" bodies 34 to x (1, 0, 0) y (0, 1, 0) z (0, 0, 1) at (0, -40, 0) in component "blades_1"
copy_body "CopyPasteBodies6'" bodies 34 makes body 35 in component "blades_1"
move_body "Move8" bodies 35 to x (1, 0, 0) y (0, 1, 0) z (0, 0, 1) at (0, -40, 0) in component "blades_1"
copy_body "CopyPasteBodies7" bodies 35 makes body 36 in component "blades_1"
move_body "Move9" bodies 36 to x (1, 0, 0) y (0, 1, 0) z (0, 0, 1) at (0, -40, 0) in component "blades_1"
sketch "Sketch5" plane through (0, 90, 0) normal (0, 1, 0) x (-1, 0, 0) in component "blades_2"
  circle A0 centre (20, 80) radius 9.795
  circle A1 centre (20, 80) radius 9.795
  constraint concentric A0 A1
extrude "Extrude4''" add sketch "Sketch5" along normal blind 16 separate body makes body 37 in component "blades_2"
combine "Combine1'" operation add target body 18 tool bodies 37 in component "blades_2"
sketch "Sketch4" plane through (0, 115, 0) normal (0, 1, 0) x (-1, 0, 0)
  circle A0 centre (-20, 80) radius 9.9
sketch "gear" plane through (0, 106, 0) normal (0, 1, 0) x (-1, 0, 0) in component "blades_2"
  circle A0 centre (20, 80) radius 9.795
  circle A1 centre (20, 80) radius 17.5
  line L0 (18.4785, 97.4337) -> (18.8145, 99.4053)
  line L1 (21.5215, 97.4337) -> (21.0167, 99.369)
  line L2 (19.7353, 101.9227) -> (20.1093, 101.9227)
  spline S0 degree 2 poles (18.8145, 99.4053) (19.2123, 101.7393) (19.7353, 101.9227) knots 0 0 0 0.277336 0.277336 0.277336 weights 1 2.508588 1
  spline S1 degree 2 poles (20.1093, 101.9227) (20.6832, 101.5066) (21.0167, 99.369) knots 0 0 0 0.278616 0.278616 0.278616 weights 1 2.778004 1
  spline S2 degree 2 poles (12.876, 98.0892) (12.5331, 100.4319) (12.9738, 100.7679) knots 0 0 0 0.277336 0.277336 0.277336 weights 1 2.508588 1
  line L3 (13.1657, 96.1103) -> (12.876, 98.0892)
  line L4 (12.9738, 100.7679) -> (13.3294, 100.8835)
  spline S3 degree 2 poles (13.3294, 100.8835) (14.0039, 100.6651) (14.9816, 98.7352) knots 0 0 0 0.278616 0.278616 0.278616 weights 1 2.778004 1
  line L5 (16.0597, 97.0506) -> (14.9816, 98.7352)
  spline S4 degree 2 poles (7.6348, 95.0024) (6.5847, 97.1245) (6.9, 97.5803) knots 0 0 0 0.277336 0.277336 0.277336 weights 1 2.508588 1
  line L6 (8.5218, 93.2099) -> (7.6348, 95.0024)
  line L7 (6.9, 97.5803) -> (7.2026, 97.8001)
  spline S5 degree 2 poles (7.2026, 97.8001) (7.9115, 97.8008) (9.4377, 96.2674) knots 0 0 0 0.278616 0.278616 0.278616 weights 1 2.778004 1
  line L8 (10.9836, 94.9985) -> (9.4377, 96.2674)
  spline S6 degree 2 poles (3.604, 90.4471) (1.9496, 92.1408) (2.1086, 92.6717) knots 0 0 0 0.277336 0.277336 0.277336 weights 1 2.508588 1
  line L9 (5.0015, 89.0164) -> (3.604, 90.4471)
  line L10 (2.1086, 92.6717) -> (2.3284, 92.9742)
  spline S7 degree 2 poles (2.3284, 92.9742) (3.0024, 93.194) (4.9278, 92.2073) knots 0 0 0 0.278616 0.278616 0.278616 weights 1 2.778004 1
  line L11 (6.7901, 91.4782) -> (4.9278, 92.2073)
  spline S8 degree 2 poles (1.1781, 84.8691) (-0.9187, 85.9687) (-0.9315, 86.5228) knots 0 0 0 0.277336 0.277336 0.277336 weights 1 2.508588 1
  line L12 (2.9494, 83.9403) -> (1.1781, 84.8691)
  line L13 (-0.9315, 86.5228) -> (-0.816, 86.8784)
  spline S9 degree 2 poles (-0.816, 86.8784) (-0.2429, 87.2957) (1.8932, 86.9523) knots 0 0 0 0.278616 0.278616 0.278616 weights 1 2.778004 1
  line L14 (3.8897, 86.8343) -> (1.8932, 86.9523)
  spline S10 degree 2 poles (0.5947, 78.8145) (-1.7393, 79.2123) (-1.9227, 79.7353) knots 0 0 0 0.277336 0.277336 0.277336 weights 1 2.508588 1
  line L15 (2.5663, 78.4785) -> (0.5947, 78.8145)
  line L16 (-1.9227, 79.7353) -> (-1.9227, 80.1093)
  spline S11 degree 2 poles (-1.9227, 80.1093) (-1.5066, 80.6832) (0.631, 81.0167) knots 0 0 0 0.278616 0.278616 0.278616 weights 1 2.778004 1
  line L17 (2.5663, 81.5215) -> (0.631, 81.0167)
  spline S12 degree 2 poles (1.9108, 72.876) (-0.4319, 72.5331) (-0.7679, 72.9738) knots 0 0 0 0.277336 0.277336 0.277336 weights 1 2.508588 1
  line L18 (3.8897, 73.1657) -> (1.9108, 72.876)
  line L19 (-0.7679, 72.9738) -> (-0.8835, 73.3294)
  spline S13 degree 2 poles (-0.8835, 73.3294) (-0.6651, 74.0039) (1.2648, 74.9816) knots 0 0 0 0.278616 0.278616 0.278616 weights 1 2.778004 1
  line L20 (2.9494, 76.0597) -> (1.2648, 74.9816)
  spline S14 degree 2 poles (4.9976, 67.6348) (2.8755, 66.5847) (2.4197, 66.9) knots 0 0 0 0.277336 0.277336 0.277336 weights 1 2.508588 1
  line L21 (6.7901, 68.5218) -> (4.9976, 67.6348)
  line L22 (2.4197, 66.9) -> (2.1999, 67.2026)
  spline S15 degree 2 poles (2.1999, 67.2026) (2.1992, 67.9115) (3.7326, 69.4377) knots 0 0 0 0.278616 0.278616 0.278616 weights 1 2.778004 1
  line L23 (5.0015, 70.9836) -> (3.7326, 69.4377)
  spline S16 degree 2 poles (9.5529, 63.604) (7.8592, 61.9496) (7.3283, 62.1086) knots 0 0 0 0.277336 0.277336 0.277336 weights 1 2.508588 1
  line L24 (10.9836, 65.0015) -> (9.5529, 63.604)
  line L25 (7.3283, 62.1086) -> (7.0258, 62.3284)
  spline S17 degree 2 poles (7.0258, 62.3284) (6.806, 63.0024) (7.7927, 64.9278) knots 0 0 0 0.278616 0.278616 0.278616 weights 1 2.778004 1
  line L26 (8.5218, 66.7901) -> (7.7927, 64.9278)
  spline S18 degree 2 poles (15.1309, 61.1781) (14.0313, 59.0813) (13.4772, 59.0685) knots 0 0 0 0.277336 0.277336 0.277336 weights 1 2.508588 1
  line L27 (16.0597, 62.9494) -> (15.1309, 61.1781)
  line L28 (13.4772, 59.0685) -> (13.1216, 59.184)
  spline S19 degree 2 poles (13.1216, 59.184) (12.7043, 59.7571) (13.0477, 61.8932) knots 0 0 0 0.278616 0.278616 0.278616 weights 1 2.778004 1
  line L29 (13.1657, 63.8897) -> (13.0477, 61.8932)
  spline S20 degree 2 poles (21.1855, 60.5947) (20.7877, 58.2607) (20.2647, 58.0773) knots 0 0 0 0.277336 0.277336 0.277336 weights 1 2.508588 1
  line L30 (21.5215, 62.5663) -> (21.1855, 60.5947)
  line L31 (20.2647, 58.0773) -> (19.8907, 58.0773)
  spline S21 degree 2 poles (19.8907, 58.0773) (19.3168, 58.4934) (18.9833, 60.631) knots 0 0 0 0.278616 0.278616 0.278616 weights 1 2.778004 1
  line L32 (18.4785, 62.5663) -> (18.9833, 60.631)
  spline S22 degree 2 poles (27.124, 61.9108) (27.4669, 59.5681) (27.0262, 59.2321) knots 0 0 0 0.277336 0.277336 0.277336 weights 1 2.508588 1
  line L33 (26.8343, 63.8897) -> (27.124, 61.9108)
  line L34 (27.0262, 59.2321) -> (26.6706, 59.1165)
  spline S23 degree 2 poles (26.6706, 59.1165) (25.9961, 59.3349) (25.0184, 61.2648) knots 0 0 0 0.278616 0.278616 0.278616 weights 1 2.778004 1
  line L35 (23.9403, 62.9494) -> (25.0184, 61.2648)
  spline S24 degree 2 poles (32.3652, 64.9976) (33.4153, 62.8755) (33.1, 62.4197) knots 0 0 0 0.277336 0.277336 0.277336 weights 1 2.508588 1
  line L36 (31.4782, 66.7901) -> (32.3652, 64.9976)
  line L37 (33.1, 62.4197) -> (32.7974, 62.1999)
  spline S25 degree 2 poles (32.7974, 62.1999) (32.0885, 62.1992) (30.5623, 63.7326) knots 0 0 0 0.278616 0.278616 0.278616 weights 1 2.778004 1
  line L38 (29.0164, 65.0015) -> (30.5623, 63.7326)
  spline S26 degree 2 poles (36.396, 69.5529) (38.0504, 67.8592) (37.8914, 67.3283) knots 0 0 0 0.277336 0.277336 0.277336 weights 1 2.508588 1
  line L39 (34.9985, 70.9836) -> (36.396, 69.5529)
  line L40 (37.8914, 67.3283) -> (37.6716, 67.0258)
  spline S27 degree 2 poles (37.6716, 67.0258) (36.9976, 66.806) (35.0722, 67.7927) knots 0 0 0 0.278616 0.278616 0.278616 weights 1 2.778004 1
  line L41 (33.2099, 68.5218) -> (35.0722, 67.7927)
  spline S28 degree 2 poles (38.8219, 75.1309) (40.9187, 74.0313) (40.9315, 73.4772) knots 0 0 0 0.277336 0.277336 0.277336 weights 1 2.508588 1
  line L42 (37.0506, 76.0597) -> (38.8219, 75.1309)
  line L43 (40.9315, 73.4772) -> (40.816, 73.1216)
  spline S29 degree 2 poles (40.816, 73.1216) (40.2429, 72.7043) (38.1068, 73.0477) knots 0 0 0 0.278616 0.278616 0.278616 weights 1 2.778004 1
  line L44 (36.1103, 73.1657) -> (38.1068, 73.0477)
  spline S30 degree 2 poles (39.4053, 81.1855) (41.7393, 80.7877) (41.9227, 80.2647) knots 0 0 0 0.277336 0.277336 0.277336 weights 1 2.508588 1
  line L45 (37.4337, 81.5215) -> (39.4053, 81.1855)
  line L46 (41.9227, 80.2647) -> (41.9227, 79.8907)
  spline S31 degree 2 poles (41.9227, 79.8907) (41.5066, 79.3168) (39.369, 78.9833) knots 0 0 0 0.278616 0.278616 0.278616 weights 1 2.778004 1
  line L47 (37.4337, 78.4785) -> (39.369, 78.9833)
  spline S32 degree 2 poles (38.0892, 87.124) (40.4319, 87.4669) (40.7679, 87.0262) knots 0 0 0 0.277336 0.277336 0.277336 weights 1 2.508588 1
  line L48 (36.1103, 86.8343) -> (38.0892, 87.124)
  line L49 (40.7679, 87.0262) -> (40.8835, 86.6706)
  spline S33 degree 2 poles (40.8835, 86.6706) (40.6651, 85.9961) (38.7352, 85.0184) knots 0 0 0 0.278616 0.278616 0.278616 weights 1 2.778004 1
  line L50 (37.0506, 83.9403) -> (38.7352, 85.0184)
  spline S34 degree 2 poles (35.0024, 92.3652) (37.1245, 93.4153) (37.5803, 93.1) knots 0 0 0 0.277336 0.277336 0.277336 weights 1 2.508588 1
  line L51 (33.2099, 91.4782) -> (35.0024, 92.3652)
  line L52 (37.5803, 93.1) -> (37.8001, 92.7974)
  spline S35 degree 2 poles (37.8001, 92.7974) (37.8008, 92.0885) (36.2674, 90.5623) knots 0 0 0 0.278616 0.278616 0.278616 weights 1 2.778004 1
  line L53 (34.9985, 89.0164) -> (36.2674, 90.5623)
  spline S36 degree 2 poles (30.4471, 96.396) (32.1408, 98.0504) (32.6717, 97.8914) knots 0 0 0 0.277336 0.277336 0.277336 weights 1 2.508588 1
  line L54 (29.0164, 94.9985) -> (30.4471, 96.396)
  line L55 (32.6717, 97.8914) -> (32.9742, 97.6716)
  spline S37 degree 2 poles (32.9742, 97.6716) (33.194, 96.9976) (32.2073, 95.0722) knots 0 0 0 0.278616 0.278616 0.278616 weights 1 2.778004 1
  line L56 (31.4782, 93.2099) -> (32.2073, 95.0722)
  spline S38 degree 2 poles (24.8691, 98.8219) (25.9687, 100.9187) (26.5228, 100.9315) knots 0 0 0 0.277336 0.277336 0.277336 weights 1 2.508588 1
  line L57 (23.9403, 97.0506) -> (24.8691, 98.8219)
  line L58 (26.5228, 100.9315) -> (26.8784, 100.816)
  spline S39 degree 2 poles (26.8784, 100.816) (27.2957, 100.2429) (26.9523, 98.1068) knots 0 0 0 0.278616 0.278616 0.278616 weights 1 2.778004 1
  line L59 (26.8343, 96.1103) -> (26.9523, 98.1068)
  dimension "d76" = 35
  dimension "d77" = 2
  dimension "d78" = 2
  dimension "d80" = 360
  constraint concentric A0 A1
  constraint coincident A1 L0.start
  constraint coincident A1 L1.start
  constraint horizontal L2
  measures "d76" diameter of A1
  measures "d77" distance of L0.start L0.end
  measures "d78" distance of L1.start L1.end
extrude "Extrude5'" add sketch "gear" against normal blind 10 separate body makes body 38 in component "blades_2"
copy_body "CopyPasteBodies2''" bodies 38 makes body 39
move_body "Move2''" bodies 39 to x (1, 0, 0) y (0, 1, 0) z (0, 0, 1) at (40, 0, 0)
copy_body "CutPasteBodies8" bodies 39 removing the originals makes body 40 in component "blades_1"
move_body "Move10" bodies 40 to x (0.819152, 0, -0.573576) y (0, 1, 0) z (0.573576, 0, 0.819152) at (-49.1027, 0, 17.9349) in component "blades_1"
move_body "Move11" bodies 40 to x (0.573576, 0, -0.819152) y (0, 1, 0) z (0.819152, 0, 0.573576) at (-59.7424, 0, 46.2525) in component "blades_1"
move_body "Move12" bodies 40 to x (1, 0, 0) y (0, 1, 0) z (0, 0, 1) at (13, 0, 3) in component "blades_1"
delete_body "RemoveBody1" bodies 40 in component "blades_1"